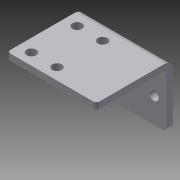
# Autodesk Inventor part: Pneumatic Piston Back Flange (Rt Custom)
Saved by Autodesk Inventor 2014 (Build 180170000, 170)
## iProperties
Created: 2014-01-13
Part Number: Pneumatic Piston Back Flange (Rt Custom)
Material: Generic
Document SubType Name: Sheet Metal
Designer: motoennies
Density: 2.71 g/cm^3
Sheet Metal Rule: Default
Appearance: Default
Flat Pattern Width: 4.445 cm
Flat Pattern Length: 6.32443 cm
Flat Pattern Area: 28.1121 cm^2
Sheet Metal Width: 1.750 in
Sheet Metal Length: 2.490 in
Sheet Metal Area: 4.357 in^2
Author: motoennies
Autodesk Inventor part; units mm, degrees
ref_plane "YZ Plane" through (0, 0, 0) normal (1, 0, 0) x (0, 1, 0)
ref_plane "XZ Plane" through (0, 0, 0) normal (0, 1, 0) x (-1, 0, 0)
ref_plane "XY Plane" through (0, 0, 0) normal (0, 0, 1) x (1, 0, 0)
sketch "Sketch1" plane through (0, 0, 0) normal (0, 0, 1) x (1, 0, 0)
  line L0 (0, 0) -> (44.45, 0)
  line L1 (44.45, 0) -> (44.45, 25.4)
  line L2 (44.45, 25.4) -> (0, 25.4)
  line L3 (0, 25.4) -> (0, 0)
  circle A0 centre (12.7, 12.7) radius 2.413
  line L4 (0, 12.7) -> (44.45, 12.7) construction
  circle A1 centre (38.1, 12.7) radius 2.413
  dimension "d0" = 44.45
  dimension "d1" = 25.4
  dimension "d2" = 4.826
  dimension "d6" = 25.4
  dimension "d32" = 6.35
  measures "d0" distance of L2.end L1.end
  measures "d1" distance of L1.end L0.end
  measures "d2" diameter of A0
  measures "d6" distance of A0.centre A1.centre
  measures "d32" distance from line of L1 A1.centre
extrude "Plate1" add sketch "Sketch1" along normal blind 3.175
sketch "Sketch2" plane through (0, 26.67, 4.445) normal (0, 1, 0) x (-1, 0, 0)
  line L0 (-44.45, 0) -> (0, 0)
  line L1 (0, 0) -> (0, 33.655)
  line L2 (0, 33.655) -> (-44.45, 33.655)
  line L3 (-44.45, 33.655) -> (-44.45, 0)
  constraints: 6 end point, 1 horizontal, 1 perpendicular, 1 vertical
edge flange "Flange1" height 38.1 angle 90 thickness 3.175 bend radius 1.27 thickness toward (0, 1, 0) relief straight relief width 3.175 relief depth 1.5875 edges at (22.225, 25.4, 3.175) wall of the first edge with corners at (44.45, 26.67, 4.445) (0, 26.67, 4.445) (0, 26.67, 38.1) (44.45, 26.67, 38.1)
bend "Bend1"
corner "Corner1"
fillet "Fillet1" radius 1.5875 4 edges at (44.45, 0, 1.5875) (0, 0, 1.5875) (0, 28.2575, 38.1) (44.45, 28.2575, 38.1)
sketch "Sketch3" plane through (0, 26.67, 4.445) normal (0, -1, 0) x (1, 0, 0)
  line L0 (3.175, 33.655) -> (22.225, 33.655) construction
  line L1 (22.225, 33.655) -> (22.225, -0.635) construction
  line L2 (22.225, -0.635) -> (3.175, -0.635) construction
  line L3 (3.175, -0.635) -> (3.175, 33.655) construction
  circle A0 centre (19.05, 27.9019) radius 2.413
  line L4 (12.7, 33.655) -> (12.7, -0.635) construction
  line L5 (3.175, 16.51) -> (22.225, 16.51) construction
  circle A1 centre (6.35, 27.9019) radius 2.413
  circle A2 centre (19.05, 5.1181) radius 2.413
  circle A3 centre (6.35, 5.1181) radius 2.413
  line L6 (44.45, 32.0675) -> (44.45, 0) projected
  line L7 (42.8625, 33.655) -> (1.5875, 33.655) projected
  point P0 (0, -4.445)
  dimension "d23" = 34.29
  dimension "d24" = 19.05
  dimension "d27" = 4.826
  dimension "d28" = 3.175
  dimension "d29" = 5.7531
  dimension "d33" = 22.225
  constraints: 12 end point, 4 centre point, 4 midpoint, 3 symmetric about line, 2 parallel, 1 collinear, 1 horizontal, 1 perpendicular, 3 other
  measures "d23" distance of L2.end L0.start
  measures "d24" distance of L0.start L0.end
  measures "d27" diameter of A0
  measures "d28" distance from line of L1 A0.centre
  measures "d29" distance from line of A0.centre L0
  measures "d33" distance between parallel lines of L6 L1
extrude "Extrusion1" cut sketch "Sketch3" against normal blind 25.4
equation "\"d12\" = BendReliefWidth"
equation "\"d13\" = BendReliefDepth"
equation "\"d14\" = MinimumRemnant"
equation "\"d15\" = BendRadius"
equation "\"d19\" = CornerReliefSize"
equation "\"d20\" = GapSize"
equation "\"d21\" = JacobiRadiusSize"
equation "\"BendRadius\" = Thickness"
equation "\"BendReliefWidth\" = Thickness"
equation "\"BendReliefDepth\" = 0.5 * Thickness"
equation "\"CornerReliefSize\" = 4 * Thickness"
equation "\"MinimumRemnant\" = 2 * Thickness"
equation "\"TransitionRadius\" = BendRadius"
equation "\"JacobiRadiusSize\" = BendRadius"
equation "\"GapSize\" = Thickness"
equation "\"d11\" = BendRadius"
equation "\"Thickness\" = 3.175"
body "Solid1"
